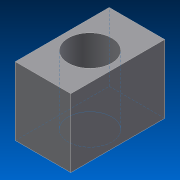
# Autodesk Inventor part: led addon
Saved by Autodesk Inventor 2015 (Build 190159000, 159)
## iProperties
Created: 2017-03-16
Part Number: led addon
Material: Generic
Document SubType Name: Modeling
Designer: ZigZagJoe
Density: 1 g/cm^3
Appearance: Default
Author: ZigZagJoe
Autodesk Inventor part; units mm, degrees
ref_plane "YZ Plane" through (0, 0, 0) normal (1, 0, 0) x (0, 1, 0)
ref_plane "XZ Plane" through (0, 0, 0) normal (0, 1, 0) x (-1, 0, 0)
ref_plane "XY Plane" through (0, 0, 0) normal (0, 0, 1) x (1, 0, 0)
sketch "Sketch1" plane through (0, 0, 0) normal (0, 0, 1) x (1, 0, 0)
  line L0 (-2.838, 7.4584) -> (3.662, 7.4584)
  line L1 (3.662, 7.4584) -> (3.662, -3.5416)
  line L2 (3.662, -3.5416) -> (-2.838, -3.5416)
  line L3 (-2.838, -3.5416) -> (-2.838, 7.4584)
  circle A0 centre (0.412, 1.9584) radius 2.55
  point P0 (0, 0)
  dimension "d0" = 5.1
  dimension "d1" = 11
  dimension "d2" = 6.5
  dimension "d3" = 3.25
  dimension "d4" = 5.5
  constraints: 8 end point, 2 parallel, 1 centre point, 1 horizontal, 1 perpendicular
  measures "d0" diameter of A0
  measures "d1" distance of L0.end L1.end
  measures "d2" distance of L1.end L2.end
  measures "d3" distance from line of L3 A0.centre
  measures "d4" distance from line of L0 A0.centre
extrude "Extrusion1" add sketch "Sketch1" along normal blind 8
equation "\"d3\" = 0.5 * d2"
equation "\"d4\" = 0.5 * d1"
body "Solid1"
